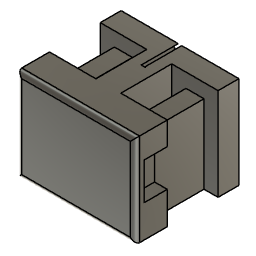
support top weight batteries (Autodesk Fusion 360 design; units mm, degrees)
Autodesk Fusion 360 part; units mm, degrees
sketch "Esquisse1" plane through (0, 0, 0) normal (0, 1, 0) x (1, 0, 0)
  line L0 (0, 0) -> (25.5, 0)
  line L1 (25.5, -20) -> (0, -20)
  line L2 (0, -20) -> (0, 0)
  line L3 (0, 0) -> (3.05, 0)
  line L4 (3.05, 0) -> (3.05, -20)
  line L5 (3.05, -20) -> (0, -20)
  line L6 (0, -20) -> (0, 0)
  line L7 (25.5, -20) -> (25.5, 0)
  line L8 (0, -20) -> (10.05, -20)
  line L9 (10.05, -20) -> (10.05, -16.95)
  line L10 (10.05, -16.95) -> (0, -16.95)
  line L11 (0, -16.95) -> (0, -20)
  line L12 (10.05, -16.95) -> (6.95, -16.95)
  line L13 (6.95, -16.95) -> (6.95, -13.85)
  line L14 (6.95, -13.85) -> (10.05, -13.85)
  line L15 (10.05, -13.85) -> (10.05, -16.95)
  line L16 (12.75, -20) -> (12.75, -6.3311)
  line L17 (15.45, -20) -> (15.45, -16.95)
  line L18 (22.45, -20) -> (25.5, -20)
  line L19 (0, -20) -> (25.5, -20)
  line L20 (15.45, -16.95) -> (25.5, -16.95)
  line L21 (22.45, 0) -> (22.45, -20)
  line L22 (25.5, -16.95) -> (25.5, -20)
  line L23 (25.5, -20) -> (25.5, 0)
  line L24 (25.5, 0) -> (22.45, 0)
  line L25 (15.45, -13.85) -> (15.45, -16.95)
  line L26 (18.55, -16.95) -> (18.55, -13.85)
  line L27 (18.55, -13.85) -> (15.45, -13.85)
  dimension "d1" = 25.5
  dimension "d2" = 20
  dimension "d3" = 3.05
  dimension "d5" = 10.05
  dimension "d6" = 3.05
  dimension "d7" = 3.1
  dimension "d8" = 3.1
  constraint horizontal L0
  constraint horizontal L1
  constraint vertical L2
  constraint coincident L0.start L2.end
  constraint horizontal L3
  constraint vertical L4
  constraint horizontal L5
  constraint vertical L6
  constraint vertical L7
  constraint horizontal L8
  constraint vertical L9
  constraint horizontal L10
  constraint vertical L11
  constraint horizontal L12
  constraint vertical L13
  constraint horizontal L14
  constraint vertical L15
  constraint midpoint L1 L16.start
  constraint perpendicular L1 L16
  constraint symmetric L1.start L16 L1.end
  constraint symmetric L1.end L16 L1.start
  constraint symmetric L0.start L16 L0.end
  constraint symmetric L3.end L16 L21.start
  constraint symmetric L4.end L16 L18.start
  constraint symmetric L8.end L16 L17.start
  constraint symmetric L9.end L16 L17.end
  constraint symmetric L10.end L16 L20.end
  constraint symmetric L12.end L16 L26.start
  constraint symmetric L13.end L16 L26.end
  constraint symmetric L14.end L16 L25.start
  measures "d1" distance of L0.start L0.end
  measures "d2" distance of L0.start L1.end
  measures "d3" distance of L0.start L3.end
  measures "d5" distance of L1.end L8.end
  measures "d6" distance of L1.end L10.end
  measures "d7" distance of L9.end L12.end
  measures "d8" distance of L9.end L14.end
extrude "Extrusion1" add sketch "Esquisse1" against normal blind 7
extrude "Extrusion3" add sketch "Esquisse1" along normal blind 15.5
extrude "Extrusion2" cut sketch "Esquisse1" along normal blind 11 contours L0 L2 L3 L4 L6 L10 | L1 L2 L4 L5 L6 L8 L10 L11 L19 | L0 L7 L20 L21 L23 L24 | L1 L4 L8 L9 L10 L12 L19 | L1 L17 L19 L20 L21 | L1 L7 L18 L19 L20 L21 L22 L23 | L10 L12 L13 L14 L15 | L20 L25 L26 L27
sketch "Esquisse2" plane through (0, -7, 0) normal (0, -1, 0) x (1, 0, 0)
  line L0 (0, 20) -> (0, 0)
  line L1 (0, 0) -> (25.5, 0)
  line L2 (25.5, 0) -> (25.5, 20)
  line L3 (25.5, 20) -> (0, 20)
  line L4 (0, 20) -> (25.5, 20)
  line L5 (25.5, 20) -> (25.5, 0)
  line L6 (25.5, 0) -> (0, 0)
  line L7 (0, 0) -> (0, 20)
  line L8 (0, 0) -> (2.75, 0)
  line L9 (2.75, 0) -> (22.75, 0)
  line L10 (22.75, 0) -> (22.75, 20)
  line L11 (22.75, 20) -> (2.75, 20)
  line L12 (2.75, 20) -> (2.75, 0)
  line L13 (2.75, 20) -> (2.75, 15)
  line L14 (2.75, 15) -> (0, 15)
  line L15 (0, 15) -> (0, 7)
  line L16 (0, 7) -> (2.75, 7)
  line L17 (2.75, 7) -> (2.75, 15)
  line L18 (12.75, 20) -> (12.75, 0)
  line L19 (22.75, 15) -> (25.5, 15)
  line L20 (25.5, 15) -> (25.5, 7)
  line L21 (22.75, 7) -> (22.75, 15)
  line L22 (25.5, 7) -> (22.75, 7)
  dimension "d15" = 20
  dimension "d16" = 25.5
  dimension "d17" = 2.75
  dimension "d18" = 20
  dimension "d19" = 5
  dimension "d20" = 8
  constraint horizontal L4
  constraint vertical L5
  constraint horizontal L6
  constraint vertical L7
  constraint coincident L1.end L2.start
  constraint coincident L0.start L3.end
  constraint coincident L0.end L1.start
  constraint perpendicular L7 L8
  constraint horizontal L9
  constraint vertical L10
  constraint horizontal L11
  constraint vertical L12
  constraint perpendicular L4 L13
  constraint horizontal L14
  constraint vertical L15
  constraint horizontal L16
  constraint vertical L17
  constraint midpoint L11 L18.start
  constraint midpoint L6 L18.end
  constraint symmetric L13.end L18 L19.start
  constraint symmetric L14.end L18 L19.end
  constraint symmetric L15.end L18 L20.end
  constraint symmetric L16.end L18 L21.start
  measures "d15" distance of L4 L6
  measures "d16" distance of L5 L7
  measures "d17" distance of L0.end L8.end
  measures "d18" distance of L8.end L9.end
  measures "d19" distance of L11.end L13.end
  measures "d20" distance of L13.end L16.end
extrude "Extrusion4" cut sketch "Esquisse2" against normal blind 7 contours L0 L7 L12 L14 L15 L16 L17 | L2 L5 L10 L19 L20 L21 L22
extrude "Extrusion5" add sketch "Esquisse2" against normal blind 2 contours L0 L7 L12 L14 L15 L16 L17 | L2 L5 L10 L19 L20 L21 L22
sketch "Esquisse3" plane through (0, 15.5, 0) normal (0, 1, 0) x (-1, 0, 0)
  line L0 (0, 0) -> (0, 20)
  line L1 (0, 20) -> (-25.5, 20)
  line L2 (-25.5, 20) -> (-25.5, 0)
  line L3 (-25.5, 0) -> (0, 0)
  line L4 (-12.75, 20) -> (-12.75, 0)
  line L5 (-12.75, 20) -> (-14.125, 20)
  line L6 (-14.125, 20) -> (-11.375, 20)
  line L7 (-11.375, 20) -> (-11.375, 10)
  line L8 (-11.375, 10) -> (-14.125, 10)
  line L9 (-14.125, 10) -> (-14.125, 20)
  line L10 (-11.375, 20) -> (-12.375, 20)
  line L11 (-11.375, 20) -> (-11.375, 19)
  line L12 (-12.375, 20) -> (-11.375, 19)
  line L13 (-11.375, 19) -> (-12.75, 19)
  line L14 (-12.375, 18) -> (-11.375, 19)
  line L15 (-12.375, 18) -> (-11.375, 18)
  line L16 (-12.375, 16) -> (-11.375, 17)
  line L17 (-12.375, 18) -> (-11.375, 17)
  line L18 (-12.375, 16) -> (-11.375, 16)
  line L19 (-12.375, 12) -> (-11.375, 13)
  line L20 (-12.375, 14) -> (-11.375, 13)
  line L21 (-12.375, 14) -> (-11.375, 15)
  line L22 (-12.375, 16) -> (-11.375, 15)
  line L23 (-12.375, 12) -> (-11.375, 12)
  line L24 (-12.375, 10) -> (-11.375, 11)
  line L25 (-12.375, 12) -> (-11.375, 11)
  line L26 (-13.125, 20) -> (-14.125, 19)
  line L27 (-13.125, 18) -> (-14.125, 19)
  line L28 (-13.125, 18) -> (-14.125, 17)
  line L29 (-13.125, 16) -> (-14.125, 17)
  line L30 (-13.125, 16) -> (-14.125, 15)
  line L31 (-13.125, 14) -> (-14.125, 15)
  line L32 (-13.125, 14) -> (-14.125, 13)
  line L33 (-13.125, 12) -> (-14.125, 13)
  line L34 (-13.125, 12) -> (-14.125, 11)
  line L35 (-13.125, 10) -> (-14.125, 11)
  dimension "d25" = 1.375
  dimension "d26" = 2.75
  dimension "d27" = 10
  dimension "d28" = 1
  dimension "d29" = 1
  constraint midpoint L1 L4.start
  constraint midpoint L3 L4.end
  constraint perpendicular L4 L5
  constraint horizontal L6
  constraint vertical L7
  constraint horizontal L8
  constraint vertical L9
  constraint perpendicular L7 L10
  constraint perpendicular L6 L11
  constraint coincident L4 L13.end
  constraint perpendicular L4 L13
  constraint symmetric L10.end L13 L14.start
  constraint symmetric L11.end L13 L12.end
  constraint coincident L7 L15.end
  constraint perpendicular L7 L15
  constraint symmetric L10.end L15 L16.start
  constraint symmetric L11.end L15 L16.end
  constraint symmetric L14.start L15 L17.start
  constraint coincident L7 L18.end
  constraint perpendicular L7 L18
  constraint symmetric L10.end L18 L19.start
  constraint symmetric L11.end L18 L19.end
  constraint symmetric L14.start L18 L20.start
  constraint symmetric L16.start L18 L22.start
  constraint symmetric L16.end L18 L21.end
  constraint coincident L7 L23.end
  constraint perpendicular L7 L23
  constraint symmetric L19.start L23 L25.start
  constraint symmetric L19.end L23 L24.end
  constraint symmetric L20.start L23 L24.start
  constraint symmetric L4 L10.end L26.start
  constraint symmetric L4 L11.end L26.end
  constraint symmetric L4 L14.start L27.start
  constraint symmetric L4 L16.start L29.start
  constraint symmetric L4 L16.end L28.end
  constraint symmetric L4 L19.start L33.start
  constraint symmetric L4 L19.end L32.end
  constraint symmetric L4 L20.start L31.start
  constraint symmetric L4 L21.end L30.end
  constraint symmetric L4 L24.start L35.start
  constraint symmetric L4 L24.end L34.end
  measures "d25" distance of L4.start L5.end
  measures "d26" distance of L5.end L6.end
  measures "d27" distance of L5.end L8.end
  measures "d28" distance of L6.end L10.end
  measures "d29" distance of L6.end L11.end
extrude "Extrusion6" cut sketch "Esquisse3" against normal blind 8 contours L1 L4 L5 L6 L8 L26 L27 L28 L29 L30 L31 L32 L33 L34 L35 | L4 L8 L13 L14 L16 L17 L19 L20 L21 L22 L24 L25 | L1 L4 L6 L12 L13
fillet "Congé1" radius 1 4 edges at (12.75, -7, 20) (25.5, -7, 10) (0, -7, 10) (12.75, -7, 0)
equation "d9 = -22.5 mm + 15.5 mm"
equation "d13 = 11 mm + 4.5 mm"
equation "d17 = ( 5.5 / 2 ) * 1 mm"
equation "d20 = 13 mm - 5 mm"
equation "d25 = ( 2.75 / 2 ) * 1 mm"
